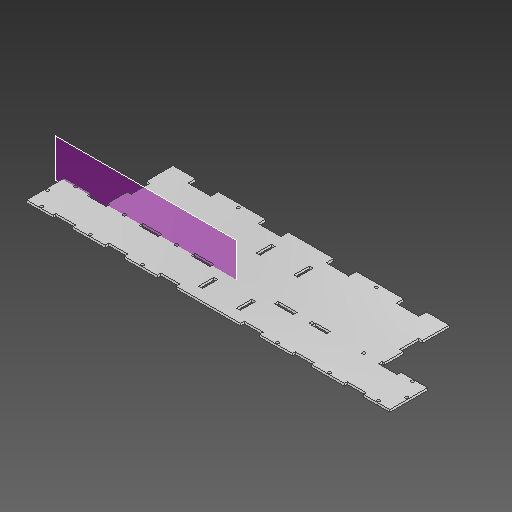
# Autodesk Inventor part: TopBottomPlates
Saved by Autodesk Inventor 2021 (Build 250183000, 183)
## iProperties
Created: 2021-03-10
Part Number: TopBottomPlates
Material: Aluminum 6061
Document SubType Name: Modeling
Designer: Dylan
Density: 2.7 g/cm^3
Appearance: Aluminum - Polished
Mass: 7184.28 g
Surface Area: 7116.28 cm^2
Volume: 2660.84 cm^3
Author: Dylan
Autodesk Inventor part; units mm, degrees
ref_plane "YZ Plane" through (0, 0, 0) normal (1, 0, 0) x (0, 1, 0)
ref_plane "XZ Plane" through (0, 0, 0) normal (0, 1, 0) x (-1, 0, 0)
ref_plane "XY Plane" through (0, 0, 0) normal (0, 0, 1) x (1, 0, 0)
sketch "Sketch1" plane through (0, 0, 0) normal (0, 1, 0) x (-1, 0, 0)
  line L0 (0, 0) -> (1219.2, 0)
  line L1 (1219.2, 0) -> (1219.2, -345.44)
  line L2 (1219.2, -345.44) -> (0, -345.44)
  line L3 (0, -345.44) -> (0, 0)
  line L4 (1219.2, -345.44) -> (1073.15, -345.44)
  line L5 (1073.15, -345.44) -> (1073.15, -152.4)
  line L6 (1073.15, -152.4) -> (1219.2, -152.4)
  line L7 (1219.2, -152.4) -> (1219.2, -345.44)
  line L8 (0, -345.44) -> (146.05, -345.44)
  line L9 (146.05, -345.44) -> (146.05, -152.4)
  line L10 (146.05, -152.4) -> (0, -152.4)
  line L11 (0, -152.4) -> (0, -345.44)
  dimension "d0" = 1219.2
  dimension "d1" = 345.44
  dimension "d3" = 152.4
  dimension "d4" = 146.05
  constraints: 24 end point, 6 parallel, 3 horizontal, 3 perpendicular, 1 collinear, 1 point on line
  measures "d0" distance of L1.end L2.end
  measures "d1" distance of L0.end L1.end
  measures "d3" distance between parallel lines of L0 L6
  measures "d4" distance of L5.end L6.end
extrude "Extrusion1" add sketch "Sketch1" along normal blind 7.9375 contours L0 L1 L6 L5 L2 L9 L10 L3
sketch "Sketch2" plane through (0, 0, 0) normal (0, -1, 0) x (1, 0, 0)
  line L0 (-51.1937, -114.3) -> (-51.1937, -127) projected
  line L1 (-37.7063, -127) -> (-51.1937, -127) projected
  line L2 (-37.7063, -114.3) -> (-37.7063, -127) projected
  line L3 (-51.1937, -114.3) -> (-37.7063, -114.3) projected
  line L4 (-214.7062, -114.3) -> (-214.7062, -127) projected
  line L5 (-201.2188, -127) -> (-214.7062, -127) projected
  line L6 (-201.2188, -114.3) -> (-201.2188, -127) projected
  line L7 (-214.7062, -114.3) -> (-201.2188, -114.3) projected
  line L8 (-384.5687, -320.04) -> (-384.5687, -345.44) projected
  line L9 (-371.0813, -345.44) -> (-384.5687, -345.44) projected
  line L10 (-371.0813, -320.04) -> (-371.0813, -345.44) projected
  line L11 (-384.5687, -320.04) -> (-371.0813, -320.04) projected
  line L12 (-848.1187, -320.04) -> (-848.1187, -345.44) projected
  line L13 (-834.6313, -345.44) -> (-848.1187, -345.44) projected
  line L14 (-834.6313, -320.04) -> (-834.6313, -345.44) projected
  line L15 (-848.1187, -320.04) -> (-834.6313, -320.04) projected
  line L16 (-1181.4937, -114.3) -> (-1181.4937, -127) projected
  line L17 (-1168.0063, -127) -> (-1181.4937, -127) projected
  line L18 (-1168.0063, -114.3) -> (-1168.0063, -127) projected
  line L19 (-1181.4937, -114.3) -> (-1168.0063, -114.3) projected
  line L20 (-1206.5, -56.7563) -> (-1219.2, -56.7563) projected
  line L21 (-1219.2, -70.2437) -> (-1219.2, -56.7563) projected
  line L22 (-1206.5, -70.2437) -> (-1219.2, -70.2437) projected
  line L23 (-1206.5, -56.7563) -> (-1206.5, -70.2437) projected
  line L24 (-1017.9812, -114.3) -> (-1017.9812, -127) projected
  line L25 (-1004.4938, -127) -> (-1017.9812, -127) projected
  line L26 (-1004.4938, -114.3) -> (-1004.4938, -127) projected
  line L27 (-1017.9812, -114.3) -> (-1004.4938, -114.3) projected
  line L28 (0, -56.7563) -> (-12.7, -56.7563) projected
  line L29 (-12.7, -70.2437) -> (-12.7, -56.7563) projected
  line L30 (0, -70.2437) -> (-12.7, -70.2437) projected
  line L31 (0, -56.7563) -> (0, -70.2437) projected
  line L32 (-375.8438, -12.7) -> (-375.8438, 0) projected
  line L33 (-389.3312, 0) -> (-375.8438, 0) projected
  line L34 (-389.3312, -12.7) -> (-389.3312, 0) projected
  line L35 (-375.8438, -12.7) -> (-389.3312, -12.7) projected
  line L36 (-949.325, 0) -> (-949.325, -12.7) projected
  line L37 (-962.025, -12.7) -> (-949.325, -12.7) projected
  line L38 (-962.025, 0) -> (-962.025, -12.7) projected
  line L39 (-949.325, 0) -> (-962.025, 0) projected
  line L40 (-1181.4937, -127) -> (-1168.0063, -114.3) construction
  line L41 (-1181.4937, -114.3) -> (-1168.0063, -127) construction
  line L42 (-1206.5, -70.2437) -> (-1219.2, -56.7563) construction
  line L43 (-1206.5, -56.7563) -> (-1219.2, -70.2437) construction
  line L44 (-962.025, -12.7) -> (-949.325, 0) construction
  line L45 (-949.325, -12.7) -> (-962.025, 0) construction
  line L46 (-848.1187, -320.04) -> (-834.6313, -345.44) construction
  line L47 (-848.1187, -345.44) -> (-834.6313, -320.04) construction
  line L48 (-375.8438, -12.7) -> (-389.3312, 0) construction
  line L49 (-389.3312, -12.7) -> (-375.8438, 0) construction
  line L50 (-214.7062, -127) -> (-201.2188, -114.3) construction
  line L51 (-214.7062, -114.3) -> (-201.2188, -127) construction
  line L52 (-51.1937, -127) -> (-37.7063, -114.3) construction
  line L53 (-51.1937, -114.3) -> (-37.7063, -127) construction
  line L54 (-12.7, -70.2437) -> (0, -56.7563) construction
  line L55 (-12.7, -56.7563) -> (0, -70.2437) construction
  line L56 (-384.5687, -345.44) -> (-371.0813, -320.04) construction
  line L57 (-384.5687, -320.04) -> (-371.0813, -345.44) construction
  line L58 (-1017.9812, -127) -> (-1004.4938, -114.3) construction
  line L59 (-1017.9812, -114.3) -> (-1004.4938, -127) construction
  line L60 (-214.7062, 0) -> (-214.7062, -12.7)
  line L61 (-201.2188, 0) -> (-201.2188, -12.7)
  line L62 (-37.7063, 0) -> (-37.7063, -12.7)
  line L63 (-1004.4938, 0) -> (-1004.4938, -12.7)
  line L64 (-1017.9812, 0) -> (-1017.9812, -12.7)
  line L65 (-1181.4937, 0) -> (-1181.4937, -12.7)
  line L66 (-1168.0063, 0) -> (-1168.0063, -12.7)
  line L67 (-1219.2, -70.2437) -> (-1206.5, -70.2437)
  line L68 (-1219.2, -56.7563) -> (-1206.5, -56.7563)
  line L69 (-1181.4937, 0) -> (-1181.4937, -12.7)
  line L70 (-1017.9812, 0) -> (-1017.9812, -12.7)
  line L71 (-1004.4938, 0) -> (-1004.4938, -12.7)
  line L72 (-843.3562, 0) -> (-843.3562, -12.7)
  line L73 (-829.8688, 0) -> (-829.8688, -12.7)
  line L74 (-389.3312, 0) -> (-389.3312, -12.7)
  line L75 (-375.8438, 0) -> (-375.8438, -12.7)
  line L76 (-214.7062, 0) -> (-214.7062, -12.7)
  line L77 (-201.2188, 0) -> (-201.2188, -12.7)
  line L78 (-37.7063, 0) -> (-37.7063, -12.7)
  line L79 (-51.1937, 0) -> (-51.1937, -12.7)
  line L80 (-1181.4937, -6.35) -> (-1168.0063, -6.35)
  line L81 (-1017.9812, -6.35) -> (-1004.4938, -6.35)
  line L82 (-843.3562, -6.35) -> (-829.8688, -6.35)
  line L83 (-214.7062, -6.35) -> (-201.2188, -6.35)
  line L84 (-51.1937, -6.35) -> (-37.7063, -6.35)
  line L85 (-836.6125, -6.35) -> (-836.6125, -120.65)
  line L86 (-836.6125, -120.65) -> (-1011.2375, -120.65)
  line L87 (-382.5875, -6.35) -> (-382.5875, -120.65)
  line L88 (-382.5875, -120.65) -> (-207.9625, -120.65)
  line L89 (-1181.4937, -127) -> (-1181.4937, -114.3)
  line L90 (-1168.0063, -127) -> (-1168.0063, -114.3)
  line L91 (-1011.2375, -6.35) -> (-1011.2375, -120.65) construction
  line L92 (-1174.75, -120.65) -> (-1174.75, -6.35) construction
  line L93 (-207.9625, -6.35) -> (-207.9625, -120.65) construction
  line L94 (-44.45, -6.35) -> (-44.45, -120.65) construction
  point P0 (0, 0)
  point P1 (-1212.85, -63.5)
  point P2 (-955.675, -6.35)
  point P3 (-841.375, -332.74)
  point P4 (-377.825, -332.74)
  point P5 (-6.35, -63.5)
  constraints: 110 end point, 25 midpoint, 22 vertical, 11 perpendicular, 8 parallel, 2 horizontal, 1 point on line, 32 other
hole "Hole1" at (-1212.85, 0, -63.5) at (-1174.75, 0, -120.65) at (-1011.2375, 0, -120.65) at (-841.375, 0, -332.74) at (-377.825, 0, -332.74) at (-207.9625, 0, -120.65) at (-44.45, 0, -120.65) at (-6.35, 0, -63.5) at (-382.5875, 0, -6.35) at (-1011.2375, 0, -6.35) at (-836.6125, 0, -6.35) at (-1174.75, 0, -6.35) at (-836.6125, 0, -120.65) at (-207.9625, 0, -6.35) at (-382.5875, 0, -120.65) at (-44.45, 0, -6.35) direction (0, 1, 0) diameter 10.0838 end through all clearance for "Hex Machine Screw" size "3/8" standard "Ansi Unified Screw Threads"
ref_plane "Work Plane1" through (-939.8, 57.15, -120.65) normal (0, 0, -1) x (-1, 0, 0)
sketch "Sketch3" plane through (0, 0, 0) normal (0, -1, 0) x (1, 0, 0)
  line L0 (-1073.15, -152.4) -> (-1219.2, -152.4) projected
  line L1 (-1219.2, -127) -> (-1073.15, -127)
  line L2 (-1073.15, -127) -> (-1073.15, -152.4)
  line L3 (-1073.15, -152.4) -> (-1219.2, -152.4)
  line L4 (-1219.2, -152.4) -> (-1219.2, -127)
  line L5 (0, 0) -> (0, -152.4) projected
  line L6 (-146.05, -152.4) -> (0, -152.4)
  line L7 (0, -152.4) -> (0, -127)
  line L8 (0, -127) -> (-146.05, -127)
  line L9 (-146.05, -127) -> (-146.05, -152.4)
  line L10 (-1219.2, 0) -> (0, 0) construction
  line L11 (-609.6, 0) -> (-609.6, -345.44) construction
  line L12 (-146.05, -345.44) -> (-1073.15, -345.44) construction
  line L13 (-1063.625, -9.525) -> (-1127.125, -9.525) projected
  line L14 (-254, -232.5359) -> (-254, -300.8619) projected
  line L15 (-88.9, -9.525) -> (-152.4, -9.525) projected
  line L16 (-263.525, -9.525) -> (-327.025, -9.525) projected
  line L17 (-955.675, -12.7) -> (-892.175, -12.7)
  line L18 (-892.175, -12.7) -> (-892.175, 0)
  line L19 (-892.175, 0) -> (-955.675, 0)
  line L20 (-955.675, 0) -> (-955.675, -12.7)
  line L21 (-781.05, -12.7) -> (-717.55, -12.7)
  line L22 (-717.55, -12.7) -> (-717.55, 0)
  line L23 (-717.55, 0) -> (-781.05, 0)
  line L24 (-781.05, 0) -> (-781.05, -12.7)
  line L25 (-666.75, -38.1) -> (-679.45, -38.1)
  line L26 (-679.45, -38.1) -> (-679.45, -88.9)
  line L27 (-679.45, -88.9) -> (-666.75, -88.9)
  line L28 (-666.75, -88.9) -> (-666.75, -38.1)
  line L29 (-892.175, -114.3) -> (-955.675, -114.3)
  line L30 (-955.675, -114.3) -> (-955.675, -127)
  line L31 (-955.675, -127) -> (-892.175, -127)
  line L32 (-892.175, -127) -> (-892.175, -114.3)
  line L33 (-1130.3, 0) -> (-1063.625, 0)
  line L34 (-1063.625, 0) -> (-1063.625, -9.525)
  line L35 (-1063.625, -9.525) -> (-1130.3, -9.525)
  line L36 (-1130.3, -9.525) -> (-1130.3, 0)
  line L37 (-1073.15, -127) -> (-1130.3, -127)
  line L38 (-1066.8, -114.3) -> (-1130.3, -114.3)
  line L39 (-1130.3, -114.3) -> (-1130.3, -127)
  line L40 (-1130.3, -127) -> (-1066.8, -127)
  line L41 (-1066.8, -127) -> (-1066.8, -114.3)
  line L42 (-1060.45, -191.77) -> (-1073.15, -191.77)
  line L43 (-1073.15, -191.77) -> (-1073.15, -255.27)
  line L44 (-1073.15, -255.27) -> (-1060.45, -255.27)
  line L45 (-1060.45, -255.27) -> (-1060.45, -191.77)
  line L46 (-920.75, -320.04) -> (-996.95, -320.04)
  line L47 (-996.95, -320.04) -> (-996.95, -345.44)
  line L48 (-996.95, -345.44) -> (-920.75, -345.44)
  line L49 (-920.75, -345.44) -> (-920.75, -320.04)
  line L50 (-685.8, -320.04) -> (-762, -320.04)
  line L51 (-762, -320.04) -> (-762, -345.44)
  line L52 (-762, -345.44) -> (-685.8, -345.44)
  line L53 (-685.8, -345.44) -> (-685.8, -320.04)
  line L54 (-666.75, -231.14) -> (-679.45, -231.14)
  line L55 (-679.45, -231.14) -> (-679.45, -281.94)
  line L56 (-679.45, -281.94) -> (-666.75, -281.94)
  line L57 (-666.75, -281.94) -> (-666.75, -231.14)
  line L58 (-501.65, -114.3) -> (-438.15, -114.3)
  line L59 (-438.15, -114.3) -> (-438.15, -127)
  line L60 (-438.15, -127) -> (-501.65, -127)
  line L61 (-501.65, -127) -> (-501.65, -114.3)
  line L62 (-375.8438, -114.3) -> (-327.025, -114.3)
  line L63 (-327.025, -114.3) -> (-327.025, -127)
  line L64 (-327.025, -127) -> (-375.8438, -127)
  line L65 (-375.8438, -127) -> (-375.8438, -114.3)
  line L66 (-152.4, -127) -> (-88.9, -127)
  line L67 (-88.9, -127) -> (-88.9, -114.3)
  line L68 (-88.9, -114.3) -> (-152.4, -114.3)
  line L69 (-152.4, -114.3) -> (-152.4, -127)
  line L70 (-152.4, -9.525) -> (-88.9, -9.525)
  line L71 (-88.9, -9.525) -> (-88.9, 0)
  line L72 (-88.9, 0) -> (-152.4, 0)
  line L73 (-152.4, 0) -> (-152.4, -9.525)
  line L74 (-263.525, -9.525) -> (-327.025, -9.525)
  line L75 (-327.025, -9.525) -> (-327.025, 0)
  line L76 (-327.025, 0) -> (-263.525, 0)
  line L77 (-263.525, 0) -> (-263.525, -9.525)
  line L78 (-438.15, 0) -> (-501.65, 0)
  line L79 (-501.65, 0) -> (-501.65, -12.7)
  line L80 (-501.65, -12.7) -> (-438.15, -12.7)
  line L81 (-438.15, -12.7) -> (-438.15, 0)
  line L82 (-539.75, -38.1) -> (-552.45, -38.1)
  line L83 (-552.45, -38.1) -> (-552.45, -88.9)
  line L84 (-552.45, -88.9) -> (-539.75, -88.9)
  line L85 (-539.75, -88.9) -> (-539.75, -38.1)
  line L86 (-539.75, -231.14) -> (-552.45, -231.14)
  line L87 (-552.45, -231.14) -> (-552.45, -281.94)
  line L88 (-552.45, -281.94) -> (-539.75, -281.94)
  line L89 (-539.75, -281.94) -> (-539.75, -231.14)
  line L90 (-457.2, -320.04) -> (-533.4, -320.04)
  line L91 (-533.4, -320.04) -> (-533.4, -345.44)
  line L92 (-533.4, -345.44) -> (-457.2, -345.44)
  line L93 (-457.2, -345.44) -> (-457.2, -320.04)
  line L94 (-222.25, -320.04) -> (-298.45, -320.04)
  line L95 (-298.45, -320.04) -> (-298.45, -345.44)
  line L96 (-298.45, -345.44) -> (-222.25, -345.44)
  line L97 (-222.25, -345.44) -> (-222.25, -320.04)
  line L98 (-158.75, -191.77) -> (-146.05, -191.77)
  line L99 (-146.05, -191.77) -> (-146.05, -255.27)
  line L100 (-146.05, -255.27) -> (-158.75, -255.27)
  line L101 (-158.75, -255.27) -> (-158.75, -191.77)
  line L102 (-781.05, -114.3) -> (-717.55, -114.3)
  line L103 (-717.55, -114.3) -> (-717.55, -127)
  line L104 (-717.55, -127) -> (-781.05, -127)
  line L105 (-781.05, -127) -> (-781.05, -114.3)
  point P0 (-1130.3, -127)
  point P1 (-263.525, -114.3)
  point P2 (-1130.3, -9.525)
  point P3 (-1219.2, -152.4)
  constraints: 196 end point, 48 parallel, 25 horizontal, 24 perpendicular, 4 point on line, 2 coincident, 1 midpoint, 1 symmetric about line, 47 other
extrude "Extrusion2" cut sketch "Sketch3" against normal through all
body "Solid1"
